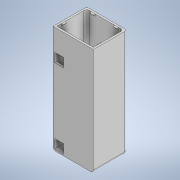
# Autodesk Inventor part: Batterihållare 2
Saved by Autodesk Inventor 2021 (Build 250183000, 183)
## iProperties
Created: 2024-12-11
Part Number: Batterihållare 2
Material: Generic
Document SubType Name: Modeling
Designer: 22liatho
Density: 1 g/cm^3
Appearance: Default
Author: 22liatho
Autodesk Inventor part; units mm, degrees
ref_plane "YZ Plane" through (0, 0, 0) normal (1, 0, 0) x (0, 1, 0)
sketch "Sketch1" plane through (0, 0, 0) normal (0, 1, 0) x (-1, 0, 0)
  line L0 (0, 0) -> (-41.2, 0)
  line L1 (-41.2, 0) -> (-41.2, -33.7)
  line L2 (-41.2, -33.7) -> (0, -33.7)
  line L3 (0, -33.7) -> (0, 0)
  line L4 (2, 2) -> (-43.2, 2)
  line L5 (-43.2, 2) -> (-43.2, -35.7)
  line L6 (-43.2, -35.7) -> (2, -35.7)
  line L7 (2, -35.7) -> (2, 2)
  dimension "d0" = 33.7
  dimension "d1" = 41.2
  dimension "d2" = 2
  dimension "d3" = 2
  dimension "d4" = 2
  dimension "d5" = 2
  constraints: 16 end point, 4 parallel, 2 horizontal, 2 perpendicular
  measures "d0" distance of L2.end L0.start
  measures "d1" distance of L1.end L2.end
  measures "d2" distance between parallel lines of L2 L6
  measures "d3" distance between parallel lines of L1 L5
  measures "d4" distance between parallel lines of L4 L0
  measures "d5" distance between parallel lines of L7 L3
extrude "Extrusion1" add sketch "Sketch1" along normal blind 2 contours L3 L2 L1 L0
extrude "Extrusion2" add sketch "Sketch1" along normal blind 120.5
sketch "Sketch2" plane through (41.2, 2, 0) normal (0, 0, -1) x (-1, 0, 0)
  line L0 (43.2, 118.5) -> (-2, 118.5) projected
  line L1 (36.2, 118.5) -> (31.2, 118.5)
  line L2 (31.2, 118.5) -> (31.2, 116.5)
  line L3 (31.2, 116.5) -> (36.2, 116.5)
  line L4 (36.2, 116.5) -> (36.2, 118.5)
  line L5 (41.2, 0) -> (41.2, 118.5) projected
  point P0 (41.2, -2)
  point P1 (31.2, 118.5)
  dimension "d10" = 5
  dimension "d11" = 2
  dimension "d12" = 5
  constraints: 8 end point, 2 parallel, 1 horizontal, 1 perpendicular, 1 point on line
  measures "d10" distance of L2.end L3.end
  measures "d11" distance of L1.end L2.end
  measures "d12" distance between parallel lines of L5 L4
sketch "Sketch3" plane through (41.2, 2, 0) normal (-1, 0, 0) x (0, 0, 1)
  point P0 (0, -2)
sketch "Sketch4" plane through (41.2, 2, 0) normal (-1, 0, 0) x (0, 0, 1)
  line L0 (2, 118.5) -> (-35.7, 118.5) projected
  line L1 (-5, 118.5) -> (-10, 118.5)
  line L2 (-10, 118.5) -> (-10, 116.5)
  line L3 (-10, 116.5) -> (-5, 116.5)
  line L4 (-5, 116.5) -> (-5, 118.5)
  line L5 (0, 0) -> (0, 118.5) projected
  point P0 (0, -2)
  dimension "d27" = 5
  dimension "d28" = 2
  dimension "d29" = 5
  constraints: 8 end point, 2 parallel, 1 horizontal, 1 perpendicular, 1 point on line
  measures "d27" distance of L2.end L3.end
  measures "d28" distance of L3.end L1.start
  measures "d29" distance between parallel lines of L5 L4
extrude "Extrusion4" add sketch "Sketch4" along normal blind 1.5
chamfer "Chamfer5" distance 0.75 distance2 1.5 1 edges at (39.7, 120.5, -7.5) measured on face at (39.7, 119.1667, -6.6667)
chamfer "Chamfer6" distance 0.75 distance2 1.5 1 edges at (39.7, 119.125, -10) measured on face at (39.7, 118.9167, -6.6667)
chamfer "Chamfer7" distance 0.75 distance2 1.5 1 edges at (39.7, 118.5, -7.1251) measured on face at (39.7, 119.3333, -7.8334)
chamfer "Chamfer8" distance 0.75 distance2 1.5 1 edges at (39.7, 119.5, -5) measured on face at (39.7, 119.5833, -6.4167)
sketch "Sketch5" plane through (0, 2, -33.7) normal (0, 0, 1) x (1, 0, 0)
  line L0 (0, 118.5) -> (41.2, 118.5) projected
  line L1 (36.2, 118.5) -> (31.2, 118.5)
  line L2 (31.2, 118.5) -> (31.2, 116.5)
  line L3 (31.2, 116.5) -> (36.2, 116.5)
  line L4 (36.2, 116.5) -> (36.2, 118.5)
  line L5 (41.2, 0) -> (41.2, 118.5) projected
  point P0 (0, -2)
  point P1 (31.2, 118.5)
  dimension "d45" = 5
  dimension "d46" = 2
  dimension "d47" = 5
  constraints: 8 end point, 2 parallel, 1 horizontal, 1 perpendicular, 1 point on line
  measures "d45" distance of L2.end L3.end
  measures "d46" distance of L1.end L2.end
  measures "d47" distance between parallel lines of L5 L4
extrude "Extrusion5" add sketch "Sketch5" along normal blind 1.5
chamfer "Chamfer9" distance 0.75 distance2 1.5 1 edges at (33.7, 120.5, -32.2) measured on face at (34.5333, 119.1667, -32.2)
chamfer "Chamfer10" distance 0.75 distance2 1.5 1 edges at (33.7, 118.5, -32.2) measured on face at (34.5333, 118.9167, -32.2)
chamfer "Chamfer11" distance 0.75 distance2 1.5 1 edges at (31.2, 119.4999, -32.2) measured on face at (34.5333, 119.4166, -32.2)
chamfer "Chamfer12" distance 0.75 distance2 1.5 1 edges at (36.2, 119.4999, -32.2) measured on face at (34.7833, 119.4166, -32.2)
ref_plane "Work Plane2" through (17.8, 0, -35.7) normal (-1, 0, 0) x (0, 0, 1)
ref_plane "Work Plane3" through (20.6, 0, 2) normal (1, 0, 0) x (0, 0, -1)
mirror "Mirror1" about plane through (20.6, 0, 2) normal (1, 0, 0) of "Extrusion5", "Extrusion4", "Chamfer5", "Chamfer8", "Chamfer7", "Chamfer9", "Chamfer11", "Chamfer10", "Chamfer12", "Chamfer6"
fillet "Fillet2" radius 3 3 edges at (-2, 0, -16.85) (20.6, 0, -35.7) (43.2, 0, -16.85)
fillet "Fillet3" radius 3 4 edges at (-1.1213, 0.8787, -34.8213) (-2, 61.75, -35.7) (42.3213, 0.8787, -34.8213) (43.2, 61.75, -35.7)
fillet "Fillet4" radius 3 2 edges at (0, 61.25, -33.7) (41.2, 61.25, -33.7)
sketch "Sketch10" plane through (-2, 120.5, 2) normal (0, 0, 1) x (1, 0, 0)
  line L0 (2, -24.4) -> (12, -24.4)
  line L1 (12, -24.4) -> (12, -34.4)
  line L2 (12, -34.4) -> (2, -34.4)
  line L3 (2, -34.4) -> (2, -24.4)
  line L4 (3, -120.5) -> (42.2, -120.5) projected
  line L5 (2, -118.5) -> (2, 0) projected
  line L6 (0, 0) -> (45.2, 0) projected
  point P0 (2, -120.5)
  dimension "d88" = 10
  dimension "d89" = 10
  dimension "d90" = 24.4
  constraints: 8 end point, 2 parallel, 1 horizontal, 1 perpendicular, 1 point on line
  measures "d88" distance of L1.end L2.end
  measures "d89" distance of L0.end L1.end
  measures "d90" distance between parallel lines of L6 L0
extrude "Extrusion10" cut sketch "Sketch10" against normal blind 10
sketch "Sketch11" plane through (-2, 120.5, 2) normal (0, 0, 1) x (1, 0, 0)
  line L0 (2, -108.5) -> (12, -108.5)
  line L1 (12, -108.5) -> (12, -118.5)
  line L2 (12, -118.5) -> (2, -118.5)
  line L3 (2, -118.5) -> (2, -108.5)
  line L4 (0, -117.5) -> (0, 0) projected
  line L5 (3, -120.5) -> (42.2, -120.5) projected
  point P0 (2, -120.5)
  dimension "d95" = 2
  dimension "d96" = 2
  dimension "d97" = 10
  dimension "d98" = 10
  constraints: 8 end point, 2 parallel, 1 horizontal, 1 perpendicular
  measures "d95" distance between parallel lines of L4 L3
  measures "d96" distance between parallel lines of L5 L2
  measures "d97" distance of L1.end L2.end
  measures "d98" distance of L0.end L1.end
extrude "Extrusion11" cut sketch "Sketch11" against normal blind 10
sketch "Sketch12" plane through (43.2, 3, 2) normal (1, 0, 0) x (0, 0, -1)
  line L0 (26.35, 103.4808) -> (11.35, 107.5)
  arc A0 (25.4441, 100.1) -> (26.35, 103.4808) centre (25.8971, 101.7904) ccw
  line L1 (25.4441, 100.1) -> (10.4441, 104.1193)
  arc A1 (11.35, 107.5) -> (10.4441, 104.1193) centre (10.8971, 105.8096) ccw
  line L2 (0, 117.5) -> (34.7, 117.5) projected
  line L3 (0, 117.5) -> (37.7, 117.5)
  line L4 (10.4441, 104.1193) -> (10.4441, 103.1193)
  line L5 (37.7, 0) -> (37.7, 117.5) projected
  line L6 (26.35, 87.9641) -> (11.35, 91.9833)
  arc A2 (25.4441, 84.5834) -> (26.35, 87.9641) centre (25.8971, 86.2737) ccw
  line L7 (25.4441, 84.5834) -> (10.4441, 88.6026)
  arc A3 (11.35, 91.9833) -> (10.4441, 88.6026) centre (10.8971, 90.293) ccw
  line L8 (10.4441, 88.6026) -> (10.4441, 87.6026)
  line L9 (26.35, 72.4474) -> (11.35, 76.4667)
  arc A4 (25.4441, 69.0667) -> (26.35, 72.4474) centre (25.8971, 70.7571) ccw
  line L10 (25.4441, 69.0667) -> (10.4441, 73.0859)
  arc A5 (11.35, 76.4667) -> (10.4441, 73.0859) centre (10.8971, 74.7763) ccw
  line L11 (10.4441, 73.0859) -> (10.4441, 72.0859)
  line L12 (26.35, 56.9308) -> (11.35, 60.95)
  arc A6 (25.4441, 53.55) -> (26.35, 56.9308) centre (25.8971, 55.2404) ccw
  line L13 (25.4441, 53.55) -> (10.4441, 57.5692)
  arc A7 (11.35, 60.95) -> (10.4441, 57.5692) centre (10.8971, 59.2596) ccw
  line L14 (10.4441, 57.5692) -> (10.4441, 56.5692)
  line L15 (26.35, 41.4141) -> (11.35, 45.4333)
  arc A8 (25.4441, 38.0333) -> (26.35, 41.4141) centre (25.8971, 39.7237) ccw
  line L16 (25.4441, 38.0333) -> (10.4441, 42.0526)
  arc A9 (11.35, 45.4333) -> (10.4441, 42.0526) centre (10.8971, 43.7429) ccw
  line L17 (10.4441, 42.0526) -> (10.4441, 41.0526)
  line L18 (26.35, 25.8974) -> (11.35, 29.9166)
  arc A10 (25.4441, 22.5167) -> (26.35, 25.8974) centre (25.8971, 24.207) ccw
  line L19 (25.4441, 22.5167) -> (10.4441, 26.5359)
  arc A11 (11.35, 29.9166) -> (10.4441, 26.5359) centre (10.8971, 28.2263) ccw
  line L20 (10.4441, 26.5359) -> (10.4441, 25.5359)
  line L21 (26.35, 10.3807) -> (11.35, 14.4)
  arc A12 (25.4441, 7) -> (26.35, 10.3807) centre (25.8971, 8.6904) ccw
  line L22 (25.4441, 7) -> (10.4441, 11.0192)
  arc A13 (11.35, 14.4) -> (10.4441, 11.0192) centre (10.8971, 12.7096) ccw
  line L23 (10.4441, 11.0192) -> (10.4441, 10.0192)
  line L24 (0, -3) -> (34.7, -3) projected
  point P0 (18.85, 105.4904)
  point P1 (18.85, 117.5)
  point P2 (18.85, 89.9737)
  point P3 (18.85, 74.457)
  point P4 (18.85, 58.9404)
  point P5 (18.85, 43.4237)
  point P6 (18.85, 27.907)
  point P7 (18.85, 12.3904)
  dimension "d113" = 15
  dimension "d114" = 3.5
  dimension "d115" = 1
  dimension "d116" = 75
  dimension "d117" = 10
  dimension "d120" = 15.5167
  dimension "d125" = 10
  constraints: 44 end point, 28 point on circle, 14 centre point, 4 tangent, 2 midpoint, 2 vertical, 1 coincident, 1 horizontal, 1 parallel, 1 vertical alignment, 78 other
  measures "d113" horizontal distance of A0.centre A1.centre
  measures "d114" distance between parallel lines of L0 L1
  measures "d115" distance of L1.end L4.end
  measures "d116" angle of L1 L4
  measures "d117" distance from line of L2 L0.end
  measures "d120" distance of L0.start L6.start
  measures "d125" distance from line of L24 L22.start
extrude "Extrusion12" [suppressed]
sketch "Sketch13" plane through (-2, 3, 2) normal (-1, 0, 0) x (0, 0, 1)
  line L0 (-9.85, 103.4808) -> (-24.85, 107.5)
  arc A0 (-10.7559, 100.1) -> (-9.85, 103.4808) centre (-10.3029, 101.7904) ccw
  line L1 (-10.7559, 100.1) -> (-25.7559, 104.1193)
  arc A1 (-24.85, 107.5) -> (-25.7559, 104.1193) centre (-25.3029, 105.8096) ccw
  line L2 (-25.7559, 104.1193) -> (-25.7559, 103.1193)
  line L3 (0, -3) -> (0, 117.5)
  line L4 (-9.85, 87.9641) -> (-24.85, 91.9833)
  arc A2 (-10.7559, 84.5834) -> (-9.85, 87.9641) centre (-10.3029, 86.2737) ccw
  line L5 (-10.7559, 84.5834) -> (-25.7559, 88.6026)
  arc A3 (-24.85, 91.9833) -> (-25.7559, 88.6026) centre (-25.3029, 90.293) ccw
  line L6 (-25.7559, 88.6026) -> (-25.7559, 87.6026)
  line L7 (-9.85, 72.4474) -> (-24.85, 76.4667)
  arc A4 (-10.7559, 69.0667) -> (-9.85, 72.4474) centre (-10.3029, 70.7571) ccw
  line L8 (-10.7559, 69.0667) -> (-25.7559, 73.0859)
  arc A5 (-24.85, 76.4667) -> (-25.7559, 73.0859) centre (-25.3029, 74.7763) ccw
  line L9 (-25.7559, 73.0859) -> (-25.7559, 72.0859)
  line L10 (-9.85, 56.9308) -> (-24.85, 60.95)
  arc A6 (-10.7559, 53.55) -> (-9.85, 56.9308) centre (-10.3029, 55.2404) ccw
  line L11 (-10.7559, 53.55) -> (-25.7559, 57.5692)
  arc A7 (-24.85, 60.95) -> (-25.7559, 57.5692) centre (-25.3029, 59.2596) ccw
  line L12 (-25.7559, 57.5692) -> (-25.7559, 56.5692)
  line L13 (-9.85, 41.4141) -> (-24.85, 45.4333)
  arc A8 (-10.7559, 38.0333) -> (-9.85, 41.4141) centre (-10.3029, 39.7237) ccw
  line L14 (-10.7559, 38.0333) -> (-25.7559, 42.0526)
  arc A9 (-24.85, 45.4333) -> (-25.7559, 42.0526) centre (-25.3029, 43.7429) ccw
  line L15 (-25.7559, 42.0526) -> (-25.7559, 41.0526)
  line L16 (-9.85, 25.8974) -> (-24.85, 29.9166)
  arc A10 (-10.7559, 22.5167) -> (-9.85, 25.8974) centre (-10.3029, 24.207) ccw
  line L17 (-10.7559, 22.5167) -> (-25.7559, 26.5359)
  arc A11 (-24.85, 29.9166) -> (-25.7559, 26.5359) centre (-25.3029, 28.2263) ccw
  line L18 (-25.7559, 26.5359) -> (-25.7559, 25.5359)
  line L19 (-9.85, 10.3807) -> (-24.85, 14.4)
  arc A12 (-10.7559, 7) -> (-9.85, 10.3807) centre (-10.3029, 8.6904) ccw
  line L20 (-10.7559, 7) -> (-25.7559, 11.0192)
  arc A13 (-24.85, 14.4) -> (-25.7559, 11.0192) centre (-25.3029, 12.7096) ccw
  line L21 (-25.7559, 11.0192) -> (-25.7559, 10.0192)
  line L22 (0, 0) -> (0, -3) projected
  line L23 (-34.7, 117.5) -> (0, 117.5) projected
  line L24 (-34.7, -3) -> (0, -3) projected
  line L25 (-37.7, 0) -> (-37.7, 117.5) projected
  line L26 (0, 0) -> (0, 117.5) projected
  line L27 (-37.7, 117.5) -> (0, 117.5)
  point P0 (-17.35, 105.4904)
  point P1 (-17.35, 89.9737)
  point P2 (-17.35, 74.457)
  point P3 (-17.35, 58.9404)
  point P4 (-17.35, 43.4237)
  point P5 (-17.35, 27.907)
  point P6 (-17.35, 12.3904)
  point P7 (-17.35, 117.5)
  dimension "d132" = 15
  dimension "d133" = 3.5
  dimension "d134" = 1
  dimension "d135" = 75
  dimension "d137" = 15.5167
  dimension "d140" = 10
  dimension "d141" = 10
  constraints: 46 end point, 28 point on circle, 14 centre point, 4 tangent, 2 midpoint, 2 vertical, 1 horizontal, 1 parallel, 1 point on line, 1 vertical alignment, 78 other
  measures "d132" horizontal distance of A0.centre A1.centre
  measures "d133" distance between parallel lines of L0 L1
  measures "d134" distance of L1.end L2.end
  measures "d135" angle of L1 L2
  measures "d137" distance of L0.start L4.start
  measures "d140" distance from line of L23 L0.end
  measures "d141" distance from line of L24 L20.start
extrude "Extrusion13" [suppressed]
body "Solid1"
